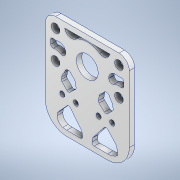
# Autodesk Inventor part: CaseSheet
Saved by Autodesk Inventor 2020.2 (Build 242310000, 310)
## iProperties
Created: 2020-01-19
Part Number: CaseSheet
Material: Aluminum 6061
Document SubType Name: Sheet Metal
Designer: Paul Lefeuvre
Density: 2.7 g/cm^3
Appearance: Aluminum - Flat
Mass: 66.3516 g
Surface Area: 151.342 cm^2
Volume: 24.5747 cm^3
Sheet Metal Rule: Default_mm
Author: Paul Lefeuvre
Autodesk Inventor part; units mm, degrees
ref_plane "YZ Plane" through (0, 0, 0) normal (1, 0, 0) x (0, 1, 0)
ref_plane "XZ Plane" through (0, 0, 0) normal (0, 1, 0) x (-1, 0, 0)
ref_plane "XY Plane" through (0, 0, 0) normal (0, 0, 1) x (1, 0, 0)
sketch "Sketch1" plane through (0, 0, 0) normal (0, 0, 1) x (1, 0, 0)
  circle A0 centre (0, 0) radius 20.6375 construction
  line L0 (-6.35, 3.6662) -> (0, 7.3323) construction
  line L1 (0, 7.3323) -> (6.35, 3.6662) construction
  line L2 (6.35, 3.6662) -> (6.35, -3.6662) construction
  line L3 (6.35, -3.6662) -> (0, -7.3323) construction
  line L4 (0, -7.3323) -> (-6.35, -3.6662) construction
  line L5 (-6.35, -3.6662) -> (-6.35, 3.6662) construction
  line L6 (0, 0) -> (0, 22.8196) construction
  line L7 (38.941, 16.1375) -> (38.941, -45.6375)
  line L8 (18.941, -65.6375) -> (-36.941, -65.6375)
  circle A1 centre (29.441, 16.1375) radius 3 construction
  circle A2 centre (29.441, 16.1375) radius 7.5 construction
  line L9 (-38.941, 16.1375) -> (-38.941, -63.6375)
  circle A3 centre (29.441, 16.1375) radius 9.5
  line L10 (29.441, 25.6375) -> (-29.441, 25.6375)
  circle A4 centre (-29.441, 16.1375) radius 3 construction
  circle A5 centre (-29.441, 16.1375) radius 9.5
  circle A6 centre (29.441, 16.1375) radius 4
  circle A7 centre (-29.441, 16.1375) radius 4
  circle A8 centre (-29.441, -10.1375) radius 3 construction
  circle A9 centre (-29.441, -10.1375) radius 10.5 construction
  circle A10 centre (-29.441, -10.1375) radius 4
  line L11 (0, -20.6375) -> (-54.2194, -20.6375) construction
  arc A11 (18.941, -65.6375) -> (38.941, -45.6375) centre (18.941, -45.6375) ccw
  circle A12 centre (0, 0) radius 7.5 construction
  arc A13 (-38.941, -63.6375) -> (-36.941, -65.6375) centre (-36.941, -63.6375) ccw
  circle A14 centre (0, 0) radius 9.5 construction
  circle A15 centre (0, 0) radius 10.1
  circle A16 centre (-29.441, -10.1375) radius 7.5 construction
  circle A17 centre (-29.441, 16.1375) radius 7.5 construction
  circle A18 centre (-29.441, -10.1375) radius 9.5 construction
  circle A19 centre (29.441, -10.1375) radius 3 construction
  circle A20 centre (29.441, -10.1375) radius 7.5 construction
  circle A21 centre (29.441, -10.1375) radius 10.5 construction
  circle A22 centre (29.441, -10.1375) radius 9.5 construction
  circle A23 centre (29.441, -10.1375) radius 4
  dimension "d0" = 41.275
  dimension "d1" = 12.7
  dimension "d3" = 65.6375
  dimension "d4" = 6
  dimension "d6" = 15
  dimension "d7" = 2
  dimension "d9" = 6
  dimension "d12" = 1
  dimension "d13" = 1
  dimension "d14" = 6
  dimension "d18" = 1
  dimension "d19" = 20
  dimension "d20" = 15
  dimension "d21" = 2
  dimension "d22" = 19
  dimension "d23" = 0.6
  dimension "d26" = 15
  dimension "d27" = 3
  dimension "d29" = 2
  dimension "d30" = 15
  dimension "d31" = 2
  dimension "d37" = 6
  dimension "d38" = 15
  dimension "d39" = 3
  dimension "d40" = 2
  dimension "d41" = 1
  dimension "d42" = 25.6375
  constraints: 24 end point, 23 centre point, 12 tangent, 10 coincident, 8 point on circle, 4 horizontal, 2 vertical, 1 perpendicular, 1 point on line, 1 vertical alignment, 17 other
  measures "d1" distance of L0.start L1.end
  measures "d3" distance from line of point (0, 0) L8
  measures "d4" diameter of A1
  measures "d6" diameter of A2
  measures "d7" radial gap between concentric circles of A2 A3
  measures "d9" diameter of A4
  measures "d12" radial gap between concentric circles of A1 A6
  measures "d13" radial gap between concentric circles of A4 A7
  measures "d14" diameter of A8
  measures "d18" radial gap between concentric circles of A8 A10
  measures "d19" radius of A11
  measures "d20" diameter of A12
  measures "d21" radius of A13
  measures "d22" diameter of A14
  measures "d23" radial gap between concentric circles of A14 A15
  measures "d26" diameter of A16
  measures "d27" radial gap between concentric circles of A9 A16
  measures "d29" radial gap between concentric circles of A5 A17
  measures "d30" diameter of A17
  measures "d31" radial gap between concentric circles of A16 A18
  measures "d37" diameter of A19
  measures "d38" diameter of A20
  measures "d39" radial gap between concentric circles of A20 A21
  measures "d40" radial gap between concentric circles of A20 A22
  measures "d41" radial gap between concentric circles of A19 A23
  measures "d42" distance from line of L10 point (0, 0)
extrude "Extrusion1" add sketch "Sketch1" along normal blind 5
sketch "Sketch2" plane through (0, 0, 5) normal (0, 0, 1) x (1, 0, 0)
  circle A0 centre (0, 0) radius 20
  circle A1 centre (29.441, 16.1375) radius 4 projected
  circle A2 centre (29.441, 16.1375) radius 9.5
  circle A3 centre (29.441, -10.1375) radius 9.5
  circle A4 centre (-29.441, 16.1375) radius 9.5
  circle A5 centre (-29.441, -10.1375) radius 9.5
  circle A6 centre (29.441, 16.1375) radius 4 projected
  circle A7 centre (-29.441, 16.1375) radius 4 projected
  circle A8 centre (-29.441, -10.1375) radius 4 projected
  circle A9 centre (29.441, -10.1375) radius 4 projected
  arc A10 (-19.9843, 0.7915) -> (-27.3195, 6.8774) centre (-25.9796, 1.0289) ccw
  arc A11 (-20.4937, 19.3304) -> (-11.4175, 16.4208) centre (-14.8427, 21.347) ccw
  arc A12 (-24.5405, -1.9991) -> (-19.9938, 0.4965) centre (-22.9929, 0.571) ccw
  arc A13 (-15.4496, -12.7008) -> (-20.5688, -13.5335) centre (-17.767, -14.6059) ccw
  arc A14 (20.5688, -13.5335) -> (15.4496, -12.7008) centre (17.767, -14.6059) ccw
  arc A15 (19.9938, 0.4965) -> (24.5405, -1.9991) centre (22.9929, 0.571) ccw
  arc A16 (27.3195, 6.8774) -> (19.9843, 0.7915) centre (25.9796, 1.0289) ccw
  arc A17 (11.4175, 16.4208) -> (20.4937, 19.3304) centre (14.8427, 21.347) ccw
  arc A18 (-29.441, 25.6375) -> (-38.941, 16.1375) centre (-29.441, 16.1375) ccw projected
  line L0 (29.441, 25.6375) -> (-29.441, 25.6375)
  line L1 (-38.941, 16.1375) -> (-38.941, -10.1375)
  line L2 (38.941, -45.6375) -> (38.941, 16.1375) projected
  line L3 (38.941, -10.1375) -> (38.941, 16.1375)
  line L4 (33.941, -1.7709) -> (33.941, 7.7709)
  line L5 (21.0744, 20.6375) -> (-21.0744, 20.6375)
  line L6 (-33.941, 7.7709) -> (-33.941, -1.7709)
  line L7 (29.3892, -56.146) -> (36.456, -16.5438)
  line L8 (-29.3891, -56.1463) -> (-36.456, -16.5438)
  line L9 (0, 40.0952) -> (0, -100.5638) construction
  line L10 (-33.941, -30.6375) -> (-33.941, -60.6375)
  line L11 (6.3999, -60.6375) -> (33.941, -60.6375)
  line L12 (33.941, -60.6375) -> (33.941, -30.6375)
  line L13 (-38.941, 16.1375) -> (-38.941, -63.6375) projected
  line L14 (-36.941, -65.6375) -> (18.941, -65.6375) projected
  arc A19 (4.4266, -58.3121) -> (6.3999, -60.6375) centre (6.3999, -58.6375) ccw
  arc A20 (-6.3999, -60.6375) -> (-4.4266, -58.3121) centre (-6.3999, -58.6375) ccw
  arc A21 (18.941, -60.6375) -> (33.941, -45.6375) centre (18.941, -45.6375) ccw
  arc A22 (-33.941, -45.6375) -> (-19.0796, -60.6375) centre (-18.9404, -45.6375) ccw
  arc A23 (-10.9918, -18.5037) -> (-12.7801, -15.384) centre (-16.0671, -19.3407) ccw
  arc A24 (12.3836, -15.705) -> (11.0927, -17.8917) centre (14.5585, -18.4633) ccw
  arc A25 (23.7668, -20.328) -> (21.9787, -16.0165) centre (15.2066, -21.3517) ccw
  arc A26 (-22.076, -16.138) -> (-23.7326, -20.0415) centre (-16.1754, -20.9454) ccw
  arc A27 (-27.664, -52.9138) -> (-22.7335, -60.1507) centre (-21.0489, -53.7049) ccw
  arc A28 (-32.8608, -51.2269) -> (-30.3932, -50.5194) centre (-31.6635, -50.7461) ccw
  line L15 (-6.3999, -60.6375) -> (-33.941, -60.6375)
  arc A29 (18.941, -65.6375) -> (38.941, -45.6375) centre (18.941, -45.6375) ccw projected
  arc A30 (-38.941, -45.6375) -> (-18.941, -65.6375) centre (-18.941, -45.6375) ccw
  line L16 (-18.941, -65.6375) -> (-38.941, -65.6375)
  line L17 (-38.941, -65.6375) -> (-38.941, -45.6375)
  line L18 (-23.4154, -23.8781) -> (-18.7877, -28.4663)
  line L19 (-12.1517, -35.9823) -> (-11.5573, -36.4518)
  line L20 (-11.0144, -23.7957) -> (-16.0078, -28.5015)
  line L21 (-21.7178, -35.2655) -> (-22.3408, -35.6443)
  line L22 (-22.0953, -31.5569) -> (-21.5647, -31.9509)
  line L23 (-15.7494, -40.9149) -> (-5.421, -53.8488)
  line L24 (-11.7285, -32.4943) -> (-12.1836, -32.8692)
  line L25 (-18.7803, -40.8047) -> (-26.8788, -49.5574)
  line L26 (-11.3247, -16.4849) -> (-10.4128, -22.0147)
  line L27 (-23.9931, -22.2203) -> (-23.4276, -17.492)
  line L28 (-28.2047, -57.4354) -> (-27.3966, -50.6782)
  line L29 (-25.3658, -33.698) -> (-25.2734, -32.9252)
  line L30 (-8.4835, -33.7126) -> (-8.3443, -34.5569)
  line L31 (-5.0105, -54.7713) -> (-4.4266, -58.3121)
  arc A31 (-12.1836, -32.8692) -> (-12.1517, -35.9823) centre (-10.912, -34.4129) ccw
  arc A32 (-21.7178, -35.2655) -> (-21.5647, -31.9509) centre (-22.757, -33.5566) ccw
  arc A33 (-18.7877, -28.4663) -> (-16.0078, -28.5015) centre (-17.3795, -27.046) ccw
  arc A34 (-15.7494, -40.9149) -> (-18.7803, -40.8047) centre (-17.3123, -42.163) ccw
  arc A35 (-23.9931, -22.2203) -> (-23.4154, -23.8781) centre (-22.0073, -22.4578) ccw
  arc A36 (-11.0144, -23.7957) -> (-10.4128, -22.0147) centre (-12.3861, -22.3402) ccw
  arc A37 (-26.8788, -49.5574) -> (-27.3966, -50.6782) centre (-25.4108, -50.9157) ccw
  arc A38 (-5.0105, -54.7713) -> (-5.421, -53.8488) centre (-6.9839, -55.0968) ccw
  line L32 (23.4154, -23.8781) -> (18.7877, -28.4663)
  line L33 (11.0144, -23.7957) -> (16.0078, -28.5015)
  line L34 (15.7494, -40.9149) -> (5.421, -53.8488)
  line L35 (18.7803, -40.8047) -> (26.8788, -49.5574)
  arc A39 (16.0078, -28.5015) -> (18.7877, -28.4663) centre (17.3795, -27.046) ccw
  arc A40 (18.7803, -40.8047) -> (15.7494, -40.9149) centre (17.3123, -42.163) ccw
  arc A41 (23.4154, -23.8781) -> (23.9931, -22.2203) centre (22.0073, -22.4578) ccw
  arc A42 (10.4128, -22.0147) -> (11.0144, -23.7957) centre (12.3861, -22.3402) ccw
  arc A43 (27.3966, -50.6782) -> (26.8788, -49.5574) centre (25.4108, -50.9157) ccw
  arc A44 (5.421, -53.8488) -> (5.0105, -54.7713) centre (6.9839, -55.0968) ccw
  line L36 (10.4128, -22.0147) -> (11.3247, -16.4849)
  line L37 (23.4276, -17.492) -> (23.9931, -22.2203)
  line L38 (4.4266, -58.3121) -> (5.0105, -54.7713)
  line L39 (27.3966, -50.6782) -> (28.2047, -57.4351)
  arc A45 (30.3932, -50.5194) -> (32.8608, -51.2269) centre (31.6635, -50.7461) ccw
  arc A46 (-22.0953, -31.5569) -> (-25.2734, -32.9252) centre (-23.2876, -33.1627) ccw
  arc A47 (-25.3658, -33.698) -> (-22.3408, -35.6443) centre (-23.38, -33.9355) ccw
  arc A48 (-11.5573, -36.4518) -> (-8.3443, -34.5569) centre (-10.3176, -34.8824) ccw
  arc A49 (-8.4835, -33.7126) -> (-11.7285, -32.4943) centre (-10.4569, -34.038) ccw
  line L40 (12.1517, -35.9823) -> (11.5573, -36.4518)
  line L41 (21.7178, -35.2655) -> (22.3408, -35.6443)
  line L42 (22.0953, -31.5569) -> (21.5647, -31.9509)
  line L43 (11.7285, -32.4943) -> (12.1836, -32.8692)
  line L44 (25.3658, -33.698) -> (25.2734, -32.9252)
  line L45 (8.4835, -33.7126) -> (8.3443, -34.5569)
  arc A50 (12.1517, -35.9823) -> (12.1836, -32.8692) centre (10.912, -34.4129) ccw
  arc A51 (21.5647, -31.9509) -> (21.7178, -35.2655) centre (22.757, -33.5566) ccw
  arc A52 (25.2734, -32.9252) -> (22.0953, -31.5569) centre (23.2876, -33.1627) ccw
  arc A53 (22.3408, -35.6443) -> (25.3658, -33.698) centre (23.38, -33.9355) ccw
  arc A54 (8.3443, -34.5569) -> (11.5573, -36.4518) centre (10.3176, -34.8824) ccw
  arc A55 (11.7285, -32.4943) -> (8.4835, -33.7126) centre (10.4569, -34.038) ccw
  arc A56 (-33.941, 1.0875) -> (-31.5063, -0.8647) centre (-31.941, 1.0875) ccw
  arc A57 (-31.5063, 6.8647) -> (-33.941, 4.9125) centre (-31.941, 4.9125) ccw
  arc A58 (33.941, 4.9125) -> (31.5063, 6.8647) centre (31.941, 4.9125) ccw
  arc A59 (31.5063, -0.8647) -> (33.941, 1.0875) centre (31.941, 1.0875) ccw
  point P0 (0, -85.153)
  point P1 (-28.5877, -60.6375)
  point P2 (28.5877, -60.6375)
  point P3 (-3.8827, -61.6103)
  point P4 (-25.8541, -37.7808)
  point P5 (-9.0485, -30.2867)
  point P6 (-7.5037, -39.6538)
  point P7 (-24.8639, -29.5012)
  point P8 (30.3932, -50.5194)
  point P9 (32.8565, -51.2375)
  dimension "d43" = 40
  dimension "d44" = 6
  dimension "d45" = 6
  dimension "d46" = 6
  dimension "d47" = 6
  dimension "d48" = 3
  dimension "d49" = 3
  dimension "d50" = 3
  dimension "d51" = 3
  dimension "d52" = 5
  dimension "d53" = 5
  dimension "d54" = 5
  dimension "d55" = 5
  dimension "d56" = 5
  dimension "d57" = 5
  dimension "d59" = 2
  dimension "d60" = 15
  dimension "d62" = 20
  dimension "d63" = 2
  dimension "d64" = 2
  dimension "d67" = 2
  dimension "d70" = 2
  dimension "d71" = 2
  dimension "d72" = 2
  dimension "d73" = 2
  constraints: 100 point on circle, 87 end point, 58 tangent, 48 centre point, 39 symmetric about line, 31 point on line, 9 equal radius, 5 vertical, 3 parallel, 2 coincident, 2 horizontal, 2 midpoint, 2 perpendicular, 93 other
  measures "d44" radius of A11
  measures "d45" radius of A17
  measures "d46" radius of A10
  measures "d47" radius of A16
  measures "d48" radius of A13
  measures "d49" radius of A12
  measures "d50" radius of A14
  measures "d51" radius of A15
  measures "d52" distance between parallel lines of L3 L4
  measures "d53" distance between parallel lines of L0 L5
  measures "d54" distance between parallel lines of L1 L6
  measures "d55" distance between parallel lines of L13 L10
  measures "d56" distance between parallel lines of L14 L11
  measures "d57" distance between parallel lines of L2 L12
  measures "d59" radius of A20
  measures "d60" radius of A21
  measures "d62" radius of A30
  measures "d63" radius of A31
  measures "d64" radius of A33
  measures "d67" radius of A46
  measures "d70" radius of A56
  measures "d71" radius of A57
  measures "d72" radius of A58
  measures "d73" radius of A59
extrude "Extrusion2" cut sketch "Sketch2" against normal blind 10 contours A0 A16 A2 A58 L4 A59 A3 A15 | A14 A3 A25 L37 A41 L32 A39 L33 A42 L36 A24 A0 | A0 A11 A4 L5 A2 A17 | A0 A12 A5 A56 L6 A57 A4 A10 | A23 L26 A36 L20 A33 L18 A35 L27 A26 A5 A13 A0 | L11 A19 L38 A44 L34 A40 L35 A43 L39 A21 | A30 L10 L15 L14 L16 L17 L13 | A30 L15 L10 | A22 A27 L28 A37 L25 A34 L23 A38 L31 A20 L15 | A31 L24 A49 L30 A48 L19 | L21 A47 L29 A46 L22 A32 | L40 A54 L45 A55 L43 A50 | A51 L42 A52 L44 A53 L41
body "Solid1"
